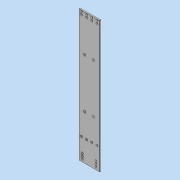
# Autodesk Inventor part: Grundgestell
Saved by Autodesk Inventor 2021 (Build 250183000, 183)
## iProperties
Created: 2024-03-15
Part Number: Grundgestell
Material: Generic
Document SubType Name: Modeling
Designer: Nokia
Density: 1 g/cm^3
Appearance: Default
Mass: 7707.64 g
Surface Area: 8625.39 cm^2
Volume: 7707.64 cm^3
Author: Nokia
Autodesk Inventor part; units mm, degrees
ref_plane "YZ Plane" through (0, 0, 0) normal (1, 0, 0) x (0, 1, 0)
ref_plane "XZ Plane" through (0, 0, 0) normal (0, 1, 0) x (-1, 0, 0)
ref_plane "XY Plane" through (0, 0, 0) normal (0, 0, 1) x (1, 0, 0)
sketch "Sketch1" plane through (0, 0, 0) normal (0, 0, 1) x (1, 0, 0)
  line L0 (0, 0) -> (-260, 0)
  line L1 (-260, 0) -> (-260, 1640)
  line L2 (-260, 1640) -> (0, 1640)
  line L3 (0, 1640) -> (0, 0)
  dimension "d0" = 260
  dimension "d1" = 1640
  constraints: 8 end point, 3 perpendicular, 1 horizontal
  measures "d0" distance of L0.start L0.end
  measures "d1" distance of L0.end L1.end
extrude "Extrusion1" add sketch "Sketch1" along normal blind 20
sketch "Sketch2" plane through (0, 0, 20) normal (0, 0, 1) x (1, 0, 0)
  line L0 (0, 1640) -> (-260, 1640) projected
  line L1 (0, 1640) -> (0, 1575)
  line L2 (0, 0) -> (0, 1640) projected
  line L3 (0, 1575) -> (-260, 1575)
  line L4 (-260, 1640) -> (-260, 0) projected
  line L5 (-260, 1607.5) -> (-260, 1640)
  line L6 (-260, 1640) -> (0, 1640)
  line L7 (-260, 1607.5) -> (0, 1607.5)
  line L8 (-130, 1623.75) -> (-65, 1623.75)
  line L9 (-130, 1640) -> (-130, 1575)
  line L10 (-65, 1640) -> (-65, 1575)
  line L11 (-97.5, 1640) -> (-97.5, 1575)
  circle A0 centre (-97.5, 1623.75) radius 7
  circle A1 centre (-32.5, 1623.75) radius 7
  circle A2 centre (-97.5, 1591.25) radius 7
  circle A3 centre (-32.5, 1591.25) radius 7
  circle A4 centre (-162.5, 1623.75) radius 7
  circle A5 centre (-227.5, 1623.75) radius 7
  circle A6 centre (-227.5, 1591.25) radius 7
  circle A7 centre (-162.5, 1591.25) radius 7
  circle A8 centre (-97.5, 1623.75) radius 14
  circle A9 centre (-32.5, 1623.75) radius 14
  circle A10 centre (-97.5, 1591.25) radius 14
  circle A11 centre (-32.5, 1591.25) radius 14
  circle A12 centre (-162.5, 1623.75) radius 14
  circle A13 centre (-227.5, 1623.75) radius 14
  circle A14 centre (-227.5, 1591.25) radius 14
  circle A15 centre (-162.5, 1591.25) radius 14
  line L12 (0, 1640) -> (0, 259)
  line L13 (0, 259) -> (-260, 259)
  line L14 (-260, 259) -> (-260, 289)
  line L15 (-130, 289) -> (0, 289)
  line L16 (-130, 289) -> (-130, 259)
  line L17 (-65, 340.0719) -> (-65, 224.44)
  line L18 (-130, 274) -> (-65, 274)
  line L19 (-97.5, 374.0039) -> (-97.5, 217.5835)
  circle A16 centre (-97.5, 274) radius 14
  circle A17 centre (-32.5, 274) radius 14
  circle A18 centre (-162.5, 274) radius 14
  circle A19 centre (-227.5, 274) radius 14
  circle A20 centre (-97.5, 274) radius 7
  circle A21 centre (-32.5, 274) radius 7
  circle A22 centre (-162.5, 274) radius 7
  circle A23 centre (-227.5, 274) radius 7
  dimension "d4" = 65
  dimension "d5" = 14
  dimension "d6" = 28
  dimension "d11" = 1381
  dimension "d12" = 30
  dimension "d13" = 28
  dimension "d14" = 14
  constraints: 34 end point, 24 centre point, 20 symmetric about line, 16 point on line, 10 perpendicular, 6 midpoint, 2 coincident, 2 vertical, 1 parallel, 20 other
  measures "d4" distance of L0.start L1.end
  measures "d5" diameter of A0
  measures "d6" diameter of A8
  measures "d11" distance of L0.start L12.end
  measures "d12" distance of L13.end L14.end
  measures "d13" diameter of A16
  measures "d14" diameter of A20
extrude "Extrusion2" cut sketch "Sketch2" against normal blind 10 contours A8 L8 A0 L11 | L11 A0 L8 A8 | A8 L11 A0 L8 | A0 L8 L11 | L11 L8 A0 | L8 A0 L11 A8 | A0 L11 L8 | A10 L11 A2 | L11 A2 A10 | L11 A0 L8 | A2 L11 | L11 A2 | A1 | A3 | A4 | A5 | A6 | A7 | A9 | A11 | A12 | A13 | A14 | A15
extrude "Extrusion3" cut sketch "Sketch2" against normal through all contours A0 L8 L11 | L11 L8 A0 | A0 L11 L8 | L11 A0 L8 | A2 L11 | L11 A2 | A1 | A3 | A4 | A5 | A6 | A7
extrude "Extrusion4" cut sketch "Sketch2" against normal through all contours A20 L18 L19 | L19 L18 A20 | A20 L19 L18 | A20 L18 L19 | A21 | A22 | A23
extrude "Extrusion5" cut sketch "Sketch2" against normal blind 10 contours A16 L18 A20 L19 | L19 A20 L18 A16 | A16 L19 A20 L18 | A16 L18 A20 L19 | A17 | A18 | A19
fillet "Fillet1" radius 4 12 edges at (-260, 820, 20) (0, 820, 20) (0, 820, 0) (-260, 820, 0) (-130, 0, 20) (-130, 0, 0) (-130, 1640, 20) (-130, 1640, 0) (0, 1640, 10) (-260, 1640, 10) (0, 0, 10) (-260, 0, 10)
sketch "Sketch3" plane through (0, 0, 20) normal (0, 0, 1) x (1, 0, 0)
  line L0 (0, 0) -> (-45.25, 0)
  line L1 (-4, 0) -> (-256, 0) projected
  line L2 (-45.25, 0) -> (-45.25, 39)
  line L3 (0, 0) -> (-130, 0)
  line L4 (-130, 0) -> (-130, 210)
  circle A0 centre (-45.25, 39) radius 13
  circle A1 centre (-45.25, 39) radius 7
  line L5 (-45.25, 39) -> (-45.25, 69)
  line L6 (-45.25, 69) -> (-45.25, 96)
  circle A2 centre (-45.25, 69) radius 13
  circle A3 centre (-45.25, 69) radius 7
  line L7 (-21, 69) -> (-25, 69)
  circle A4 centre (-45.25, 99) radius 13
  circle A5 centre (-45.25, 99) radius 7
  circle A6 centre (-214.75, 39) radius 13
  circle A7 centre (-214.75, 39) radius 7
  circle A8 centre (-214.75, 69) radius 13
  circle A9 centre (-214.75, 69) radius 7
  circle A10 centre (-214.75, 99) radius 13
  circle A11 centre (-214.75, 99) radius 7
  dimension "d20" = 45.25
  dimension "d21" = 39
  dimension "d22" = 26
  dimension "d23" = 14
  dimension "d24" = 30
  dimension "d25" = 27
  dimension "d26" = 14
  constraints: 14 end point, 12 centre point, 8 coincident, 8 symmetric about line, 3 vertical, 2 point on line, 1 horizontal, 1 midpoint, 8 other
  measures "d20" distance of L0.start L0.end
  measures "d21" distance of L0.end L2.end
  measures "d22" diameter of A0
  measures "d23" diameter of A1
  measures "d24" distance of L5.start L5.end
  measures "d25" distance of L5.end L6.end
  measures "d26" diameter of A3
extrude "Extrusion6" cut sketch "Sketch3" against normal blind 14.5
extrude "Extrusion7" cut sketch "Sketch3" against normal through all contours A1 L5 L2 | L2 L5 A1 | A3 L6 L5 | L5 L6 A3 | A5 | A7 | A9 | A11
sketch "Sketch4" plane through (0, 0, 0) normal (0, 0, -1) x (-1, 0, 0)
  circle A0 centre (75, 1178.75) radius 14
  circle A1 centre (185, 1178.75) radius 14
  circle A2 centre (185, 563.75) radius 14
  circle A3 centre (75, 563.75) radius 14
  constraints: 4 centre point
extrude "Extrusion8" cut sketch "Sketch4" against normal through all
body "Solid1"
